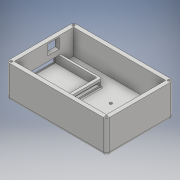
# Autodesk Inventor part: Back Plate test08
Saved by Autodesk Inventor 2018.3 (Build 223285000, 285)
## iProperties
Created: 2022-01-10
Part Number: Back Plate test08
Material: Generic
Document SubType Name: Modeling
Designer: Stewart Alexander
Density: 1 g/cm^3
Appearance: Default
Author: Stewart Alexander
Autodesk Inventor part; units mm, degrees
ref_plane "YZ Plane" through (0, 0, 0) normal (1, 0, 0) x (0, 1, 0)
ref_plane "XZ Plane" through (0, 0, 0) normal (0, 1, 0) x (-1, 0, 0)
ref_plane "XY Plane" through (0, 0, 0) normal (0, 0, 1) x (1, 0, 0)
sketch "Arduino Uno" plane through (0, 0, 0) normal (0, 0, 1) x (1, 0, 0)
  line L0 (0, 0) -> (68.6, 0)
  line L1 (68.6, 0) -> (68.6, 53.3)
  line L2 (68.6, 53.3) -> (0, 53.3)
  line L3 (0, 53.3) -> (0, 0)
  circle A0 centre (14, 2.5) radius 1.6
  circle A1 centre (66.1, 7.6) radius 1.6
  circle A2 centre (66.1, 35.5) radius 1.6
  circle A3 centre (15.3, 50.7) radius 1.6
  dimension "d97" = 68.6
  dimension "d98" = 53.3
  dimension "d99" = 3.2
  dimension "d100" = 2.5
  dimension "d101" = 14
  dimension "d102" = 3.2
  dimension "d103" = 66.1
  dimension "d104" = 7.6
  dimension "d105" = 3.2
  dimension "d106" = 35.5
  dimension "d107" = 66.1
  dimension "d108" = 3.2
  dimension "d109" = 15.3
  dimension "d110" = 50.7
  constraints: 8 end point, 4 centre point, 2 parallel, 1 horizontal, 1 perpendicular
  measures "d97" distance of L2.end L1.end
  measures "d98" distance of L0.end L1.end
  measures "d99" diameter of A0
  measures "d100" vertical distance of L0.start A0.centre
  measures "d101" horizontal distance of L0.start A0.centre
  measures "d102" diameter of A1
  measures "d103" horizontal distance of L0.start A1.centre
  measures "d104" vertical distance of L0.start A1.centre
  measures "d105" diameter of A2
  measures "d106" vertical distance of L0.start A2.centre
  measures "d107" horizontal distance of L0.start A2.centre
  measures "d108" diameter of A3
  measures "d109" horizontal distance of L0.start A3.centre
  measures "d110" vertical distance of L0.start A3.centre
sketch "Sketch2" plane through (0, 0, 0) normal (0, 0, 1) x (1, 0, 0)
  line L0 (-7.6136, -10.2044) -> (-7.6136, 63.0956)
  line L1 (-7.6136, 63.0956) -> (106.3864, 63.0956)
  line L2 (106.3864, 63.0956) -> (106.3864, -10.2044)
  line L3 (106.3864, -10.2044) -> (-7.6136, -10.2044)
  dimension "d29" = 114
  dimension "d39" = 73.3
  constraints: 8 end point, 3 perpendicular
  measures "d29" distance of L0.end L1.end
  measures "d39" distance of L0.start L0.end
extrude "Back Plate" add sketch "Sketch2" against normal blind 10
extrude "Uno Mounting Holes" cut sketch "Arduino Uno" against normal blind 7 contours A0 | A1 | A2 | A3
sketch "3.5\" TFT LCD Screen" plane through (0, 0, 0) normal (0, 0, 1) x (1, 0, 0)
  line L0 (88.6005, 0.0003) -> (88.6005, 53.3003)
  line L1 (88.6005, 53.3003) -> (10.6005, 53.3003)
  line L2 (10.6005, 53.3003) -> (10.6005, 0.0003)
  line L3 (10.6005, 0.0003) -> (88.6005, 0.0003)
  line L4 (-7.6136, -10.2044) -> (-7.6136, 63.0956) projected
  line L5 (106.3864, -10.2044) -> (-7.6136, -10.2044) projected
  line L6 (106.3864, 63.0956) -> (106.3864, -10.2044) projected
  line L7 (-7.6136, 63.0956) -> (106.3864, 63.0956) projected
  point P0 (0, 0)
  point P1 (68.6, 0)
  dimension "d35" = 78
  dimension "d36" = 53.3
  dimension "d37" = 78
  dimension "d38" = 53.3
  constraints: 8 end point
  measures "d35" distance of L2.end L0.start
  measures "d36" distance of L1.end L2.end
  measures "d37" distance of L0.end L1.end
  measures "d38" distance of L0.start L0.end
sketch "SD Card Slot" plane through (0, 0, 0) normal (0, 0, 1) x (1, 0, 0)
  line L0 (39.3864, 9.1) -> (-7.6136, 9.1)
  line L1 (-7.6136, 9.1) -> (-7.6136, 44.1)
  line L2 (-7.6136, 44.1) -> (39.3864, 44.1)
  line L3 (39.3864, 44.1) -> (39.3864, 9.1)
  circle A0 centre (14, 2.5) radius 1.6 projected
  line L4 (-7.6136, -10.2044) -> (-7.6136, 63.0956) projected
  circle A1 centre (15.3, 50.7) radius 1.6 projected
  point P0 (0, 0)
  dimension "d41" = 35
  dimension "d42" = 47
  dimension "d44" = 6.6
  dimension "d45" = 0
  constraints: 8 end point, 2 parallel, 1 horizontal, 1 perpendicular
  measures "d41" distance of L0.end L1.end
  measures "d42" distance of L0.start L0.end
  measures "d44" distance from line of L0 A0.centre
  measures "d45" distance between parallel lines of L4 L1
sketch "Sketch5" plane through (0, 0, 0) normal (0, 0, 1) x (1, 0, 0)
  line L0 (39.3864, 9.1) -> (-7.6136, 9.1) projected
  line L1 (39.3864, 44.1) -> (39.3864, 9.1) projected
  line L2 (-7.6136, 44.1) -> (39.3864, 44.1) projected
  line L3 (-7.6136, 9.1) -> (-7.6136, 44.1) projected
  line L4 (39.8864, 8.6) -> (39.8864, 44.6)
  line L5 (39.8864, 8.6) -> (-7.6136, 8.6)
  line L6 (-7.6136, -10.2044) -> (-7.6136, 63.0956) projected
  line L7 (39.8864, 44.6) -> (-7.6136, 44.6)
  line L8 (-7.6136, 44.6) -> (-7.6136, 47.1)
  line L9 (-7.6136, 47.1) -> (43.3864, 47.1)
  line L10 (-7.6136, 8.6) -> (-7.6136, 6.1)
  line L11 (-7.6136, 6.1) -> (43.3864, 6.1)
  line L12 (43.3864, 6.1) -> (43.3864, 47.1)
  point P0 (0, 0)
  dimension "d47" = 2.5
  dimension "d48" = 51
  dimension "d49" = 2.5
  dimension "d72" = 0.5
  dimension "d73" = 0.5
  dimension "d74" = 0.5
  constraints: 16 end point, 4 perpendicular, 3 point on line, 1 horizontal, 1 parallel
  measures "d47" distance of L7.end L8.end
  measures "d48" distance of L8.end L9.end
  measures "d49" distance of L5.end L10.end
  measures "d72" distance between parallel lines of L1 L4
  measures "d73" distance between parallel lines of L0 L5
  measures "d74" distance between parallel lines of L2 L7
extrude "SD Card Slot Slot" add sketch "Sketch5" along normal blind 10 contours L5 L4 L7 L6 L9 L12 L11
sketch "Sketch6" plane through (43.3864, 6.1, 0) normal (1, 0, 0) x (0, 0, -1)
  line L0 (0, 41) -> (0, 0) projected
  line L1 (0, 41) -> (-10, 41) projected
  line L2 (-10, 0) -> (-10, 41) projected
  line L3 (0, 0) -> (-10, 0) projected
  line L4 (-7, 38) -> (-3, 38)
  line L5 (-3, 38) -> (-3, 3)
  line L6 (-3, 3) -> (-7, 3)
  line L7 (-7, 3) -> (-7, 38)
  point P0 (0, -6.1)
  dimension "d52" = 3
  constraints: 8 end point, 3 other
  measures "d52" distance between parallel lines of L2 L7
extrude "SD Ribbon Slot" cut sketch "Sketch6" against normal through all contours L4 L5 L6 L7
fillet "1.2mm Fillet" radius 1.2 7 edges at (17.8864, 47.1, 0) (17.8864, 6.1, 0) (43.3864, 26.6, 0) (43.3864, 6.1, 5) (43.3864, 47.1, 5) (39.8864, 44.6, 5) (39.8864, 8.6, 5)
sketch "Sketch7" plane through (0, 0, 0) normal (0, 0, 1) x (1, 0, 0)
  line L0 (106.3864, -10.2044) -> (101.3864, -10.2044)
  line L1 (101.3864, -10.2044) -> (101.3864, -5.2044)
  line L2 (101.3864, -5.2044) -> (106.3864, -5.2044)
  line L3 (106.3864, -5.2044) -> (106.3864, -10.2044)
  line L4 (49.3864, -10.2044) -> (49.3864, 80.0118)
  line L5 (-7.6136, 63.0956) -> (106.3864, 63.0956) projected
  line L6 (106.3864, 26.4456) -> (-34.6963, 26.4456)
  line L7 (-7.6136, -10.2044) -> (-2.6136, -10.2044)
  line L8 (-2.6136, -10.2044) -> (-2.6136, -5.2044)
  line L9 (-2.6136, -5.2044) -> (-7.6136, -5.2044)
  line L10 (-7.6136, -5.2044) -> (-7.6136, -10.2044)
  line L11 (106.3864, 63.0956) -> (101.3864, 63.0956)
  line L12 (101.3864, 63.0956) -> (101.3864, 58.0956)
  line L13 (101.3864, 58.0956) -> (106.3864, 58.0956)
  line L14 (106.3864, 58.0956) -> (106.3864, 63.0956)
  line L15 (-7.6136, 63.0956) -> (-2.6136, 63.0956)
  line L16 (-2.6136, 63.0956) -> (-2.6136, 58.0956)
  line L17 (-2.6136, 58.0956) -> (-7.6136, 58.0956)
  line L18 (-7.6136, 58.0956) -> (-7.6136, 63.0956)
  point P0 (0, 0)
  point P1 (0, 52.8913)
  dimension "d56" = 5
  dimension "d57" = 5
  dimension "d58" = 57
  dimension "d59" = 36.65
  constraints: 36 end point, 11 symmetric about line, 2 parallel, 2 perpendicular, 1 horizontal
  measures "d56" distance of L1.end L2.end
  measures "d57" distance of L0.end L1.end
  measures "d58" distance of L0.start L4.start
  measures "d59" distance of L0.start L6.start
extrude "Pillars" [suppressed]
sketch "Sketch8" plane through (0, 0, 31) normal (0, 0, 1) x (1, 0, 0)
  line L0 (101.3864, -10.2044) -> (-2.6136, -10.2044) projected
  line L1 (-7.6136, -5.2044) -> (-2.6136, -5.2044) projected
  line L2 (101.3864, -10.2044) -> (-2.6136, -10.2044)
  line L3 (-2.6136, -10.2044) -> (-2.6136, -5.2044)
  line L4 (-2.6136, -5.2044) -> (101.3864, -5.2044)
  line L5 (101.3864, -5.2044) -> (101.3864, -10.2044)
  line L6 (101.3864, 63.0956) -> (101.3864, 58.0956) projected
  line L7 (106.3864, 63.0956) -> (106.3864, -10.2044) projected
  line L8 (101.3864, 58.0956) -> (106.3864, 58.0956)
  line L9 (106.3864, 58.0956) -> (106.3864, -5.2044)
  line L10 (106.3864, -5.2044) -> (101.3864, -5.2044)
  line L11 (101.3864, -5.2044) -> (101.3864, 58.0956)
  line L12 (-7.6136, 58.0956) -> (-2.6136, 58.0956) projected
  line L13 (-7.6136, 63.0956) -> (106.3864, 63.0956) projected
  line L14 (-2.6136, 58.0956) -> (101.3864, 58.0956)
  line L15 (101.3864, 58.0956) -> (101.3864, 63.0956)
  line L16 (101.3864, 63.0956) -> (-2.6136, 63.0956)
  line L17 (-2.6136, 63.0956) -> (-2.6136, 58.0956)
  line L18 (-2.6136, 58.0956) -> (-7.6136, 58.0956)
  line L19 (-7.6136, 58.0956) -> (-7.6136, -5.2044)
  line L20 (-7.6136, -5.2044) -> (-2.6136, -5.2044)
  line L21 (-2.6136, -5.2044) -> (-2.6136, 58.0956)
  point P0 (0, 0)
  constraints: 32 end point, 8 parallel, 4 horizontal, 4 perpendicular, 3 point on line
extrude "Beams (Will they print?)" [suppressed]
sketch "Sketch9" plane through (0, 0, 0) normal (0, 0, 1) x (1, 0, 0)
  line L0 (106.3864, 63.0956) -> (106.3864, -10.2044) projected
  line L1 (-7.6136, -10.2044) -> (-7.6136, 63.0956) projected
  line L2 (106.3864, -10.2044) -> (-7.6136, -10.2044)
  line L3 (-7.6136, -10.2044) -> (-7.6136, 63.0956)
  line L4 (-7.6136, 63.0956) -> (106.3864, 63.0956) projected
  line L5 (-7.6136, 63.0956) -> (106.3864, 63.0956)
  line L6 (106.3864, 63.0956) -> (106.3864, -10.2044)
  line L7 (106.3864, -10.2044) -> (106.3864, -15.2044)
  line L8 (106.3864, -15.2044) -> (-7.6136, -15.2044)
  line L9 (-7.6136, -15.2044) -> (-12.6136, -15.2044)
  line L10 (-12.6136, -15.2044) -> (-12.6136, 63.0956)
  line L11 (-12.6136, 63.0956) -> (-12.6136, 68.0956)
  line L12 (-12.6136, 68.0956) -> (106.3864, 68.0956)
  line L13 (106.3864, 68.0956) -> (111.3864, 68.0956)
  line L14 (111.3864, 68.0956) -> (111.3864, -15.2044)
  line L15 (111.3864, -15.2044) -> (106.3864, -15.2044)
  point P0 (0, 0)
  dimension "d64" = 5
  dimension "d65" = 5
  dimension "d66" = 5
  dimension "d67" = 5
  constraints: 26 end point, 8 point on line, 6 perpendicular, 2 collinear, 1 horizontal
  measures "d64" distance of L0.end L7.end
  measures "d65" distance of L8.end L9.end
  measures "d66" distance of L10.end L11.end
  measures "d67" distance of L12.end L13.end
extrude "Outer Walls (5mm Offset)" add sketch "Sketch9" along normal blind 31 and the other way blind 10
extrude "Extrusion9" [suppressed]
sketch "Sketch10" plane through (-12.6136, -15.2044, 31) normal (-1, 0, 0) x (0, 0, 1)
  line L0 (-31, 58.6044) -> (-21, 58.6044) projected
  line L1 (-29.8, 61.1044) -> (-29.8, 22.5044) projected
  line L2 (-21, 58.6044) -> (-21, 25.0044) projected
  line L3 (-21, 58.6044) -> (-21, 25.0044)
  line L4 (-21, 25.0044) -> (-29.8, 25.0044)
  line L5 (-29.8, 25.0044) -> (-29.8, 58.6044)
  line L6 (-29.8, 58.6044) -> (-21, 58.6044)
  line L7 (-31, 63.5044) -> (-31, 78.3) projected
  line L8 (-13.6, 59.5047) -> (-2.9, 59.5047)
  line L9 (-2.9, 59.5047) -> (-2.9, 47.5047)
  line L10 (-2.9, 47.5047) -> (-13.6, 47.5047)
  line L11 (-13.6, 47.5047) -> (-13.6, 59.5047)
  line L12 (-1.9, 46.5047) -> (-1.9, 60.5047)
  line L13 (-1.9, 60.5047) -> (-14.6, 60.5047)
  line L14 (-14.6, 60.5047) -> (-14.6, 46.5047)
  line L15 (-14.6, 46.5047) -> (-1.9, 46.5047)
  point P0 (-31, 15.2044)
  point P1 (-31, 68.5047)
  point P2 (-21, 59.8044)
  point P3 (-21, 23.8044)
  dimension "d82" = 10.7
  dimension "d83" = 12
  dimension "d84" = 1
  constraints: 24 end point, 7 perpendicular, 3 point on line, 2 collinear, 1 horizontal, 3 other
  measures "d82" distance of L8.start L8.end
  measures "d83" distance of L8.end L9.end
  measures "d84" distance between parallel lines of L9 L12
extrude "SD Card Opening" cut sketch "Sketch10" against normal blind 5 contours L0 L2 L4 L1 | L8 L9 L10 L11 | L15 L14 L13 L12
fillet "4mm Fillet" radius 4 8 edges at (-12.6136, 68.0956, 10.5) (-12.6136, -15.2044, 10.5) (111.3864, -15.2044, 10.5) (111.3864, 68.0956, 10.5) (49.3864, 68.0956, -10) (-12.6136, 26.4456, -10) (49.3864, -15.2044, -10) (111.3864, 26.4456, -10)
sketch "Sketch11" plane through (0, 0, 0) normal (0, 0, 1) x (1, 0, 0)
  line L0 (98.4778, 47.4456) -> (98.4778, 5.4456) construction
  line L1 (98.4778, 5.4456) -> (86.054, 5.4456) construction
  line L2 (86.054, 5.4456) -> (86.054, 47.4456) construction
  line L3 (86.054, 47.4456) -> (98.4778, 47.4456) construction
  line L4 (-8.6136, 68.0956) -> (107.3864, 68.0956) projected
  line L5 (107.3864, 68.0956) -> (107.3864, 26.4456)
  line L6 (107.3864, 26.4456) -> (48.9636, 26.4456)
  point P0 (0, 0)
  dimension "d88" = 41.65
  dimension "d89" = 42
  dimension "d90" = 21
  constraints: 4 end point, 1 perpendicular, 1 vertical, 2 other
  measures "d88" distance of L4.end L5.end
  measures "d89" distance of L1.end L2.end
  measures "d90" distance between parallel lines of L6 L3
feature "Inside Text" [suppressed]
sketch "Sketch12" plane through (0, 0, 31) normal (0, 0, 1) x (1, 0, 0)
  circle A0 centre (108.3864, -12.2044) radius 1.5
  line L0 (-12.6136, -15.2044) -> (111.3864, -15.2044) projected
  line L1 (111.3864, -15.2044) -> (111.3864, 68.0956) projected
  line L2 (107.3864, -15.2044) -> (-8.6136, -15.2044) projected
  line L3 (49.3864, -15.2044) -> (49.3864, 77.1219)
  line L4 (-8.6136, -11.2044) -> (-12.6136, -11.2044) projected
  line L5 (-12.6136, -11.2044) -> (-12.6136, 26.4456)
  line L6 (-12.6136, -11.2044) -> (-12.6136, 64.0956) projected
  line L7 (-12.6136, 26.4456) -> (133.0429, 26.4456)
  circle A1 centre (-9.6136, -12.2044) radius 1.5
  line L8 (111.3864, 26.4456) -> (-34.2702, 26.4456)
  circle A2 centre (108.3864, 65.0956) radius 1.5
  line L9 (-8.6136, 64.0956) -> (-12.6136, 64.0956)
  circle A3 centre (-9.6136, 65.0956) radius 1.5
  point P0 (0, 0)
  point P1 (111.3864, -11.2044)
  point P2 (111.3864, 64.0956)
  dimension "d91" = 3
  dimension "d92" = 3
  dimension "d93" = 3
  dimension "d94" = 37.65
  constraints: 10 end point, 6 symmetric about line, 4 centre point, 2 midpoint, 2 perpendicular, 3 other
  measures "d91" diameter of A0
  measures "d92" distance from line of L0 A0.centre
  measures "d93" distance from line of L1 A0.centre
  measures "d94" distance of L4.end L5.end
extrude "3mm Screw Holes" cut sketch "Sketch12" against normal blind 15 contours A0 | A1 | A2 | A3
sketch "Sketch13" plane through (-7.6136, 8.6, 0) normal (1, 0, 0) x (0, 0, -1)
  line L0 (-10, 1.2) -> (-10, 0)
  line L1 (-10, 0) -> (0, 0)
  line L2 (0, 0) -> (0, 36) projected
  line L3 (0, 0) -> (0, 36)
  line L4 (0, 36) -> (-10, 36)
  line L5 (-10, 34.8) -> (-1.2, 34.8) projected
  line L6 (-10, 36) -> (-10, 34.8)
  line L7 (-10, 34.8) -> (-1.2, 34.8)
  line L8 (-1.2, 34.8) -> (-1.2, 1.2) projected
  line L9 (-1.2, 34.8) -> (-1.2, 1.2)
  line L10 (-1.2, 1.2) -> (-10, 1.2) projected
  line L11 (-1.2, 1.2) -> (-10, 1.2)
  point P0 (0, -8.6)
  constraints: 16 end point, 4 perpendicular, 3 collinear, 1 vertical
extrude "Extrusion11" cut sketch "Sketch13" against normal blind 4
body "Solid1"
